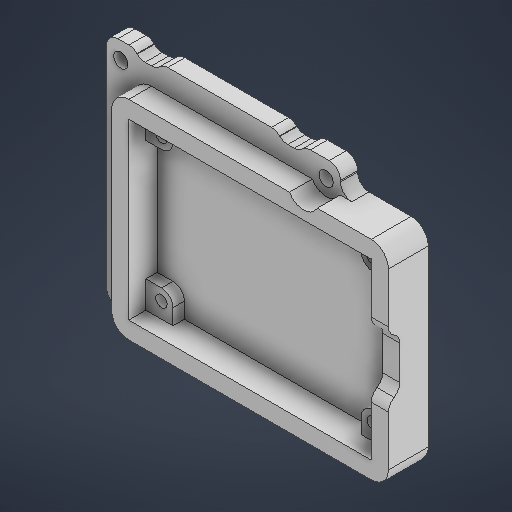
# Autodesk Inventor part: 陀螺仪外壳2
Saved by Autodesk Inventor 2025 (Build 290162000, 162)
## iProperties
Created: 2025-01-04
Part Number: 陀螺仪外壳2
Material: 常规
Document SubType Name: Modeling
Designer: HZD
Density: 1 g/cm^3
Appearance: 默认
Author: HZD
Autodesk Inventor part; units mm, degrees
ref_plane "YZ Plane" through (0, 0, 0) normal (1, 0, 0) x (0, 1, 0)
ref_plane "XZ Plane" through (0, 0, 0) normal (0, 1, 0) x (-1, 0, 0)
ref_plane "XY Plane" through (0, 0, 0) normal (0, 0, 1) x (1, 0, 0)
sketch "草图1" plane through (0, 0, 0) normal (0, 0, 1) x (1, 0, 0)
  line L0 (21.25, -15.25) -> (-21.25, -15.25)
  line L1 (-21.25, -15.25) -> (-21.25, 15.25)
  line L2 (-21.25, 15.25) -> (21.25, 15.25)
  line L3 (21.25, 15.25) -> (21.25, -15.25)
  line L4 (21.25, -15.25) -> (-21.25, 15.25) construction
  line L5 (-21.25, -15.25) -> (21.25, 15.25) construction
  line L6 (24.25, -18.25) -> (-24.25, -18.25)
  line L7 (-24.25, -18.25) -> (-24.25, 18.25)
  line L8 (-24.25, 18.25) -> (24.25, 18.25)
  line L9 (24.25, 18.25) -> (24.25, -18.25)
  point P0 (0, 0)
  dimension "d0" = 42.5
  dimension "d1" = 30.5
  dimension "d2" = 3
  constraints: 20 end point, 4 parallel, 2 midpoint, 2 perpendicular, 1 horizontal, 3 other
  measures "d0" distance of L1.end L2.end
  measures "d1" distance of L0.end L1.end
  measures "d2" distance between parallel lines of L3 L9
extrude "拉伸1" add sketch "草图1" along normal blind 2 contours L0 L1 L2 L3 | L6 L7 L8 L9
extrude "拉伸2" add sketch "草图1" along normal blind 7
fillet "圆角1" radius 3 4 edges at (24.25, 18.25, 3.5) (-24.25, 18.25, 3.5) (-24.25, -18.25, 3.5) (24.25, -18.25, 3.5)
sketch "草图2" plane through (0, 0, 2) normal (0, 0, 1) x (1, 0, 0)
  circle A0 centre (-18.5, 12.5) radius 1
  line L0 (21.25, 18.25) -> (-21.25, 18.25) projected
  line L1 (0, 18.25) -> (0, 0)
  line L2 (-24.25, 15.25) -> (-24.25, -15.25) projected
  line L3 (-24.25, 0) -> (0, 0)
  circle A1 centre (-18.5, 12.5) radius 2
  line L4 (-16.5, 12.5) -> (-16.5, 15.8598)
  line L5 (-16.5, 15.8598) -> (-22.5422, 15.8598)
  line L6 (-22.5422, 15.8598) -> (-22.5422, 10.5)
  line L7 (-22.5422, 10.5) -> (-18.5, 10.5)
  dimension "d8" = 2
  dimension "d9" = 18.5
  dimension "d10" = 12.5
  dimension "d11" = 4
  constraints: 12 end point, 3 perpendicular, 2 centre point, 2 midpoint, 2 point on circle, 2 vertical, 1 coincident, 1 tangent
  measures "d8" diameter of A0
  measures "d9" distance from line of A0.centre L1
  measures "d10" distance from line of L3 A0.centre
  measures "d11" diameter of A1
extrude "拉伸3" add sketch "草图2" along normal blind 2
extrude "拉伸4" cut sketch "草图2" against normal blind 4 contours A0
mirror "镜像1" about plane through (0, 0, 0) normal (1, 0, 0) of "拉伸4", "拉伸3"
mirror "镜像2" about plane through (0, 0, 0) normal (0, 1, 0) of "拉伸3", "拉伸4", "镜像1"
sketch "草图3" plane through (0, 0, 0) normal (-1, 0, 0) x (0, -1, 0)
  point P0 (0, 0)
sketch "草图4" plane through (24.25, -15.25, 0) normal (1, 0, 0) x (0, 0, -1)
  line L0 (-5, 10.25) -> (-19.7194, 10.25)
  line L1 (-19.7194, 10.25) -> (-19.7194, 20.25)
  line L2 (-19.7194, 20.25) -> (-5, 20.25)
  line L3 (-5, 20.25) -> (-5, 10.25)
  line L4 (-5, 10.25) -> (-19.7194, 20.25) construction
  line L5 (-19.7194, 10.25) -> (-5, 20.25) construction
  line L6 (-5, 4.75) -> (-5, 25.75)
  line L7 (0, 15.25) -> (-12.1154, 15.25)
  line L8 (0, 0) -> (0, 30.5) projected
  line L9 (-7, 0) -> (-7, 30.5) projected
  point P0 (-12.3597, 15.25)
  dimension "d16" = 10
  dimension "d20" = 2
  constraints: 16 end point, 2 midpoint, 2 parallel, 2 perpendicular, 1 collinear, 1 horizontal, 1 point on line
  measures "d16" distance of L0.end L1.end
  measures "d20" distance between parallel lines of L3 L9
extrude "拉伸5" cut sketch "草图4" against normal blind 4
fillet "圆角2" radius 2 4 edges at (22.75, 5, 7) (22.75, -5, 7) (22.75, 5, 5) (22.75, -5, 5)
sketch "草图5" plane through (0, 0, 0) normal (0, 0, -1) x (-1, 0, 0)
  point P0 (0, 0)
sketch "草图7" plane through (0, 0, 0) normal (0, 0, -1) x (-1, 0, 0)
  circle A0 centre (26.629, -16.4911) radius 1.2499 projected
  circle A1 centre (26.6416, 19.5088) radius 1.2499 projected
  circle A2 centre (-9.3583, 19.5214) radius 1.2499 projected
  line L0 (29.1449, -18.25) -> (-11.8551, -18.25)
  line L1 (-11.8551, -18.25) -> (-11.8551, 22.5007)
  line L2 (-11.8551, 22.5007) -> (29.1449, 22.5007)
  line L3 (29.1449, 22.5007) -> (29.1449, -18.25)
  line L4 (29.1449, -23.9378) -> (29.1449, -19.438) projected
  line L5 (21.25, -18.25) -> (-21.25, -18.25) projected
  line L6 (-11.8551, -27.6778) -> (-11.8551, 30.5222) projected
  circle A3 centre (-18.5, -12.5) radius 1 projected
  circle A4 centre (18.5, -12.5) radius 1 projected
  circle A5 centre (-18.5, 12.5) radius 1 projected
  circle A6 centre (18.5, 12.5) radius 1 projected
  arc A7 (-24.25, -15.25) -> (-21.25, -18.25) centre (-21.25, -15.25) ccw projected
  line L7 (21.25, -18.25) -> (-21.25, -18.25) projected
  arc A8 (21.25, -18.25) -> (24.25, -15.25) centre (21.25, -15.25) ccw projected
  line L8 (24.25, 15.25) -> (24.25, -15.25) projected
  arc A9 (24.25, 15.25) -> (21.25, 18.25) centre (21.25, 15.25) ccw projected
  line L9 (-21.25, 18.25) -> (21.25, 18.25) projected
  arc A10 (-21.25, 18.25) -> (-24.25, 15.25) centre (-21.25, 15.25) ccw projected
  line L10 (-24.25, -15.25) -> (-24.25, 15.25) projected
  point P0 (0, 0)
  point P1 (-11.8551, 18.25)
  constraints: 8 end point, 3 collinear, 2 parallel, 1 horizontal, 1 perpendicular
extrude "拉伸7" add sketch "草图7" against normal blind 3 contours L0 A8 L8 A9 L9 L1 L2 L3
sketch "草图8" plane through (0, 0, 3) normal (0, 0, 1) x (1, 0, 0)
  circle A0 centre (9.3583, 19.5214) radius 1.2499 projected
  circle A1 centre (9.3583, 19.5214) radius 2.7499
  point P0 (0, 0)
  dimension "d28" = 1.5
  constraints: 1 centre point
  measures "d28" radial gap between concentric circles of A0 A1
extrude "拉伸8" cut sketch "草图8" along normal blind 8 contours A0 | A1
fillet "圆角6" radius 2 4 edges at (11.8551, 22.5007, 1.5) (11.8551, 18.25, 1.5) (-29.1449, 22.5007, 1.5) (-29.1449, -18.25, 1.5)
sketch "草图9" plane through (0, 0, 3) normal (0, 0, 1) x (1, 0, 0)
  line L0 (-24.4124, 22.8098) -> (-24.4152, 30.8098) projected
  line L1 (-19.2152, 30.8116) -> (-19.2124, 22.8116) projected
  arc A0 (-20.7119, 21.3111) -> (-19.2124, 22.8116) centre (-21.8128, 23.9107) ccw projected
  line L2 (-20.7119, 21.3111) -> (-22.9119, 21.3103) projected
  arc A1 (-24.4124, 22.8098) -> (-22.9119, 21.3103) centre (-21.8128, 23.9107) ccw projected
  line L3 (-23.7155, 31.51) -> (-19.9155, 31.5113) projected
  arc A2 (-23.7155, 31.51) -> (-24.4152, 30.8098) centre (-23.7152, 30.81) ccw projected
  arc A3 (-19.2152, 30.8116) -> (-19.9155, 31.5113) centre (-19.9152, 30.8113) ccw projected
  line L4 (1.2743, 31.5185) -> (5.0743, 31.5199) projected
  arc A4 (5.7745, 30.8201) -> (5.0743, 31.5199) centre (5.0745, 30.8199) ccw projected
  line L5 (5.7745, 30.8201) -> (5.7773, 22.8201) projected
  line L6 (0.5773, 22.8183) -> (0.5745, 30.8183) projected
  arc A5 (1.2743, 31.5185) -> (0.5745, 30.8183) centre (1.2745, 30.8185) ccw projected
  arc A6 (0.5773, 22.8183) -> (2.0778, 21.3188) centre (3.1769, 23.9192) ccw projected
  line L7 (4.2778, 21.3196) -> (2.0778, 21.3188) projected
  arc A7 (4.2778, 21.3196) -> (5.7773, 22.8201) centre (3.1769, 23.9192) ccw projected
  point P0 (0, 0)
extrude "拉伸9" cut sketch "草图9" against normal blind 8
fillet "圆角7" radius 2 8 edges at (0.736, 22.5007, 1.5) (2.0778, 21.3188, 1.5) (4.2778, 21.3196, 1.5) (5.6178, 22.5007, 1.5) (-22.9119, 21.3103, 1.5) (-20.7119, 21.3111, 1.5) (-19.367, 22.5007, 1.5) (-24.2586, 22.5007, 1.5)
ref_plane "工作平面1" through (0, 0, 0) normal (1, 0, 0) x (0, 1, 0)
ref_plane "工作平面2" through (0, 0, 0) normal (-1, 0, 0) x (0, -1, 0)
ref_plane "工作平面3" through (0, 0, 0) normal (-1, 0, 0) x (0, -1, 0)
equation "\"d14\" = d11"
equation "\"d17\" = d11"
